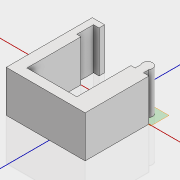
# Autodesk Inventor part: ЛЦМК.30000.10.00.03 Крышка передняя
Saved by Autodesk Inventor 2021.2 (Build 252289000, 289)
## iProperties
Created: 2025-11-22
Part Number: ЛЦМК.30000.10.00.03 Крышка передняя
Material: Типовые
Document SubType Name: Modeling
Designer: Захаров
Density: 1 g/cm^3
Appearance: По умолчанию
Author: Захаров
Autodesk Inventor part; units mm, degrees
ref_plane "YZ Plane" through (0, 0, 0) normal (1, 0, 0) x (0, 1, 0)
ref_plane "XZ Plane" through (0, 0, 0) normal (0, 1, 0) x (-1, 0, 0)
ref_plane "XY Plane" through (0, 0, 0) normal (0, 0, 1) x (1, 0, 0)
ref_plane "РабПлоскость1" through (-13, -63, -6) normal (0, -1, 0) x (1, 0, 0)
sketch "Эскиз1" plane through (-13, -63, -6) normal (0, -1, 0) x (1, 0, 0)
  arc A0 (21, 4) -> (24, 4) centre (22.5, 3.005) ccw projected
  line L0 (21, 4) -> (21, 6) projected
  line L1 (24, 6) -> (24, 4) projected
  line L2 (23.9, 6) -> (23.9, 3.9694)
  arc A1 (21.1, 3.9694) -> (23.9, 3.9694) centre (22.5, 3.005) ccw
  line L3 (21.1, 3.9694) -> (21.1, 6)
  line L4 (24, 6) -> (26, 6) projected
  line L5 (17, 6) -> (21, 6) projected
  line L6 (19.5, 4) -> (19.5, 25.5) projected
  line L7 (19.5, 25.5) -> (1.5, 25.5) projected
  line L8 (1.5, 25.5) -> (1.5, 4) projected
  line L9 (0, 6) -> (4, 6) projected
  line L10 (0, 0) -> (0, 6) projected
  line L11 (26, 6) -> (26, 29)
  line L12 (26, 29) -> (-2.4303, 29)
  line L13 (-2.4303, 29) -> (-2.4303, -2)
  line L14 (-2.4303, -2) -> (2, -2)
  line L15 (2, -2) -> (2, 0)
  line L16 (0, 0) -> (2, 0)
  point P0 (13, 6)
  point P1 (1.5, 6)
  point P2 (19.5, 6)
  dimension "d0" = 0.1
  dimension "d1" = 23
  dimension "d2" = 2
  dimension "d3" = 2
  constraints: 16 end point, 4 perpendicular, 2 point on circle, 1 centre point, 1 horizontal, 1 vertical, 2 other
  measures "d0" radial gap between concentric circles of A0 A1
  measures "d1" distance of L4.end L11.end
  measures "d2" vertical distance of L13.end L10.start
  measures "d3" horizontal distance of L14.end L10.start
extrude "Выдавливание1" add sketch "Эскиз1" against normal blind 15
fillet "Сопряжение1" radius 2 8 edges at (-15.4303, -55.5, -8) (-15.4303, -63, 7.5) (-15.4303, -48, 7.5) (-15.4303, -55.5, 23) (-1.2151, -63, 23) (-1.2151, -48, 23) (13, -63, 11.5) (13, -48, 11.5)
